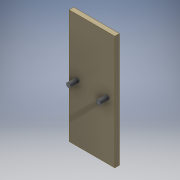
# Autodesk Inventor part: BasePlate
Saved by Autodesk Inventor 2018.1 (Build 221151000, 151)
## iProperties
Created: 2012-05-31
Part Number: BasePlate
Material: Generic
Document SubType Name: Modeling
Designer: normanpa
Density: 1 g/cm^3
Appearance: Default
Author: normanpa
Autodesk Inventor part; units mm, degrees
ref_plane "YZ Plane" through (0, 0, 0) normal (1, 0, 0) x (0, 1, 0)
ref_plane "XZ Plane" through (0, 0, 0) normal (0, 1, 0) x (-1, 0, 0)
ref_plane "XY Plane" through (0, 0, 0) normal (0, 0, 1) x (1, 0, 0)
sketch "Sketch1" plane through (0, 0, 0) normal (0, 0, 1) x (1, 0, 0)
  line L0 (-25.4, -63.5) -> (25.4, -63.5)
  line L1 (25.4, -63.5) -> (25.4, 63.5)
  line L2 (25.4, 63.5) -> (-25.4, 63.5)
  line L3 (-25.4, 63.5) -> (-25.4, -63.5)
  line L4 (-25.4, -63.5) -> (25.4, 63.5) construction
  line L5 (25.4, -63.5) -> (-25.4, 63.5) construction
  point P0 (0, 0)
  dimension "d0" = 50.8
  dimension "d2" = 127
  constraints: 12 end point, 2 midpoint, 2 parallel, 1 horizontal, 1 perpendicular
  measures "d0" distance of L1.end L2.end
  measures "d2" distance of L0.end L1.end
extrude "Extrusion1" add sketch "Sketch1" against normal blind 5.08
sketch "Sketch2" plane through (0, 0, 0) normal (0, 0, 1) x (1, 0, 0)
  circle A0 centre (16.637, 0) radius 2.3876
  circle A1 centre (-16.637, 0) radius 2.3876
  point P0 (0, 0)
  dimension "d5" = 4.7752
  dimension "d8" = 33.274
  dimension "d9" = 16.637
  constraints: 2 centre point, 1 equal radius, 1 horizontal alignment
  measures "d5" diameter of A1
  measures "d8" distance of A0.centre A1.centre
  measures "d9" distance of A0.centre point (0, 0)
extrude "Extrusion2" add sketch "Sketch2" along normal blind 9.525 separate body
thread "Thread1" size "10-24 UNC" class "2A" standard "ANSI Unified Screw Threads" full length
thread "Thread2" size "10-24 UNC" class "2A" standard "ANSI Unified Screw Threads" full length
equation "\"d9\" = 0.5 * d8"
